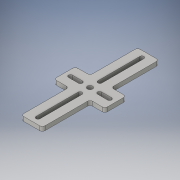
# Autodesk Inventor part: inertiabar
Saved by Autodesk Inventor 2016 (Build 200138000, 138)
## iProperties
Created: 2017-06-16
Part Number: inertiabar
Material: Generic
Document SubType Name: Modeling
Designer: Kyle
Density: 1 g/cm^3
Appearance: Default
Author: Kyle
Autodesk Inventor part; units mm, degrees
ref_plane "YZ Plane" through (0, 0, 0) normal (1, 0, 0) x (0, 1, 0)
ref_plane "XZ Plane" through (0, 0, 0) normal (0, 1, 0) x (-1, 0, 0)
ref_plane "XY Plane" through (0, 0, 0) normal (0, 0, 1) x (1, 0, 0)
sketch "Sketch1" plane through (0, 0, 0) normal (0, 1, 0) x (-1, 0, 0)
  line L0 (-12.7, 69.85) -> (12.7, 69.85)
  line L1 (12.7, -69.85) -> (-12.7, -69.85)
  line L2 (-12.7, 69.85) -> (12.7, -69.85) construction
  line L3 (12.7, 69.85) -> (-12.7, -69.85) construction
  line L4 (30.48, 12.7) -> (30.48, -12.7)
  line L5 (-30.48, -12.7) -> (-30.48, 12.7)
  line L6 (-30.48, 12.7) -> (30.48, -12.7) construction
  line L7 (30.48, 12.7) -> (-30.48, -12.7) construction
  circle A0 centre (0, 0) radius 3.175
  line L8 (0, 64.77) -> (0, 9.525) construction
  line L9 (-2.413, 62.357) -> (-2.413, 11.938)
  line L10 (2.413, 11.938) -> (2.413, 62.357)
  arc A1 (2.413, 62.357) -> (-2.413, 62.357) centre (0, 62.357) ccw
  arc A2 (-2.413, 11.938) -> (2.413, 11.938) centre (0, 11.938) ccw
  line L11 (25.908, 0) -> (9.017, 0) construction
  line L12 (23.495, 2.413) -> (11.43, 2.413)
  line L13 (11.43, -2.413) -> (23.495, -2.413)
  arc A3 (23.495, -2.413) -> (23.495, 2.413) centre (23.495, 0) ccw
  arc A4 (11.43, 2.413) -> (11.43, -2.413) centre (11.43, 0) ccw
  line L14 (-2.413, -62.357) -> (-2.413, -11.938)
  line L15 (2.413, -11.938) -> (2.413, -62.357)
  arc A5 (-2.413, -62.357) -> (2.413, -62.357) centre (0, -62.357) ccw
  arc A6 (2.413, -11.938) -> (-2.413, -11.938) centre (0, -11.938) ccw
  line L16 (-23.495, 2.413) -> (-11.43, 2.413)
  line L17 (-11.43, -2.413) -> (-23.495, -2.413)
  arc A7 (-23.495, 2.413) -> (-23.495, -2.413) centre (-23.495, 0) ccw
  arc A8 (-11.43, -2.413) -> (-11.43, 2.413) centre (-11.43, 0) ccw
  line L18 (12.7, 12.7) -> (30.48, 12.7)
  line L19 (12.7, 69.85) -> (12.7, 12.7)
  line L20 (12.7, -12.7) -> (12.7, -69.85)
  line L21 (-12.7, -12.7) -> (-30.48, -12.7)
  line L22 (30.48, -12.7) -> (12.7, -12.7)
  line L23 (-30.48, 12.7) -> (-12.7, 12.7)
  line L24 (-12.7, 12.7) -> (-12.7, 69.85)
  line L25 (-12.7, -69.85) -> (-12.7, -12.7)
  point P0 (0, 37.1475)
  point P1 (17.4625, 0)
  dimension "d0" = 25.4
  dimension "d1" = 139.7
  dimension "d2" = 60.96
  dimension "d3" = 25.4
  dimension "d4" = 6.35
  dimension "d5" = 4.826
  dimension "d6" = 4.826
  dimension "d7" = 5.08
  dimension "d8" = 9.525
  dimension "d9" = 4.572
  dimension "d10" = 9.017
  constraints: 56 end point, 20 point on circle, 16 parallel, 12 symmetric about line, 9 centre point, 9 midpoint, 8 tangent, 5 perpendicular, 4 point on line, 3 horizontal, 1 coincident, 1 horizontal alignment, 1 vertical, 1 vertical alignment, 4 other
  measures "d0" distance of L1.start L1.end
  measures "d1" distance of L0.end L1.start
  measures "d2" distance of L4.end L5.start
  measures "d3" distance of L4.start L4.end
  measures "d4" diameter of A0
  measures "d5" diameter of A2
  measures "d6" diameter of A4
  measures "d7" distance from line of L0 L8.start
  measures "d8" distance of A0.centre L8.end
  measures "d9" distance from line of L4 L11.start
  measures "d10" distance of point (0, 0) L11.end
extrude "Extrusion1" add sketch "Sketch1" along normal blind 5.08
fillet "Fillet1" radius 3.175 12 edges at (12.7, 2.54, 69.85) (-12.7, 2.54, 69.85) (12.7, 2.54, 12.7) (30.48, 2.54, 12.7) (30.48, 2.54, -12.7) (12.7, 2.54, -12.7) (-12.7, 2.54, -12.7) (-12.7, 2.54, 12.7) (-30.48, 2.54, 12.7) (-30.48, 2.54, -12.7) (-12.7, 2.54, -69.85) (12.7, 2.54, -69.85)
body "Solid1"
